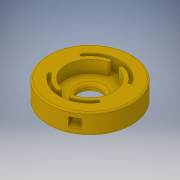
# Autodesk Inventor part: BasePaletas
Saved by Autodesk Inventor 2019 (Build 230136000, 136)
## iProperties
Created: 2019-12-12
Part Number: BasePaletas
Material: Generic
Document SubType Name: Modeling
Designer: Sergio
Density: 1 g/cm^3
Appearance: Gold
Author: Sergio
Autodesk Inventor part; units mm, degrees
ref_plane "XZ Plane" through (0, 0, 0) normal (0, 1, 0) x (-1, 0, 0)
sketch "Sketch3" plane through (0, 0, 0) normal (1, 0, 0) x (0, 1, 0)
  line L0 (63.5252, 0) -> (0, 0) construction
  line L1 (0, -7) -> (0, -27)
  line L2 (0, -27) -> (13, -27)
  line L3 (13, -27) -> (13, -15.23)
  line L4 (0, -7) -> (5, -7)
  line L5 (5, -7) -> (5, -15.23)
  line L6 (5, -15.23) -> (13, -15.23)
  dimension "d15" = 13
  dimension "d18" = 5
  dimension "d28" = 7
  dimension "d32" = 27
  dimension "d33" = 15.23
  constraints: 14 end point, 3 perpendicular, 2 horizontal, 1 coincident, 1 parallel, 1 vertical
  measures "d15" distance between parallel lines of L3 L1
  measures "d18" distance of L1.start L4.end
  measures "d28" distance between parallel lines of L4 L0
  measures "d32" distance between parallel lines of L0 L2
  measures "d33" distance between parallel lines of L0 L6
revolve "Revolution1" add sketch "Sketch3" angle 360 about axis through (0, 63.5252, 0) along (0, -1, 0)
fillet "Fillet2" radius 1 2 edges at (0, 13, 27) (0, 0, 27)
ref_plane "Work Plane2" through (-27, 6.5, 0) normal (1, 0, 0) x (0, 1, 0)
sketch "Sketch4" plane through (-27, 6.5, 0) normal (1, 0, 0) x (0, 1, 0)
  line L0 (-6.5, 0) -> (13.3256, 0) construction
  line L1 (-3.0202, 3.035) -> (3.0498, 3.035)
  line L2 (3.0498, 3.035) -> (3.0498, -3.035)
  line L3 (3.0498, -3.035) -> (-3.0202, -3.035)
  line L4 (-3.0202, -3.035) -> (-3.0202, 3.035)
  line L5 (-3.0202, 3.035) -> (3.0498, -3.035) construction
  line L6 (3.0498, 3.035) -> (-3.0202, -3.035) construction
  point P0 (0.0148, 0)
  dimension "d21" = 6.07
  dimension "d22" = 6.07
  constraints: 14 end point, 2 horizontal, 2 midpoint, 2 parallel, 1 perpendicular, 1 point on line
  measures "d21" distance of L2.end L3.end
  measures "d22" distance of L1.end L2.end
extrude "Extrusion3" cut sketch "Sketch4" along normal blind 10
pattern_circular "Circular Pattern2" count 3 over 360 about axis through (0, 9, 0) along (0, -1, 0) of "Extrusion3"
fillet "Fillet4" radius 2 1 edges at (0, 0, 7)
fillet "Fillet5" radius 2 1 edges at (0, 5, 7)
ref_plane "Work Plane3" through (0, 6.5, -27) normal (0, 0, 1) x (1, 0, 0)
sketch "Sketch5" plane through (0, 6.5, -27) normal (0, 0, 1) x (1, 0, 0)
  line L0 (27, 5.5) -> (-27, 5.5) projected
  line L1 (-3.7766, 5.5) -> (3.7234, 5.5)
  line L2 (3.7234, 5.5) -> (3.7234, 3.9)
  line L3 (3.7234, 3.9) -> (-3.7766, 3.9)
  line L4 (-3.7766, 3.9) -> (-3.7766, 5.5)
  line L5 (-0.0266, 2.2373) -> (-0.0266, 10.6054) construction
  point P0 (0, -6.5)
  dimension "d34" = 3.75
  dimension "d35" = 3.75
  dimension "d36" = 1.6
  constraints: 10 end point, 2 parallel, 1 horizontal, 1 perpendicular, 1 point on line, 1 vertical
  measures "d34" distance between parallel lines of L2 L5
  measures "d35" distance between parallel lines of L4 L5
  measures "d36" distance of L3.end L1.start
extrude "Extrusion4" cut sketch "Sketch5" along normal blind 7
sketch "Sketch7" plane through (0, 13, 0) normal (0, 1, 0) x (1, 0, 0)
  arc A0 (-13.8497, -9.3315) -> (13.8497, -9.3315) centre (0, 0) ccw
  arc A1 (-3.0841, -11.7521) -> (3.0841, -11.7521) centre (0, 0) ccw
  line L0 (0, 33.2339) -> (0, -33.2339) construction
  circle A2 centre (0, 0) radius 13.45 construction
  circle A3 centre (0, 0) radius 15.7 construction
  arc A4 (-3.3691, -14.3087) -> (-3.0841, -11.7521) centre (-3.4141, -13.0095) ccw
  arc A5 (3.0841, -11.7521) -> (3.7441, -14.2669) centre (3.4141, -13.0095) ccw
  arc A6 (-12.191, -8.2139) -> (-13.8497, -9.3315) centre (-13.0204, -8.7727) ccw
  arc A7 (13.8497, -9.3315) -> (12.399, -7.9891) centre (13.0204, -8.7727) ccw
  arc A8 (-12.191, -8.2139) -> (-3.3691, -14.3087) centre (0, 0) ccw
  arc A9 (3.7441, -14.2669) -> (12.399, -7.9891) centre (0, 0) ccw
  point P0 (0, 0)
  dimension "d42" = 26.9
  dimension "d43" = 31.4
  dimension "d40" = 33.4
  dimension "d41" = 24.3
  constraints: 16 point on circle, 8 centre point, 5 coincident, 2 end point, 2 symmetric about line, 1 tangent, 1 vertical, 8 other
  measures "d40" diameter of A0
  measures "d41" diameter of A1
sketch "Sketch8" plane through (0, 13, 0) normal (0, 1, 0) x (1, 0, 0)
  line L0 (0, 33.2339) -> (0, -33.2339) construction
  circle A0 centre (0, 0) radius 16.45 construction
  circle A1 centre (0, 0) radius 18.7 construction
  circle A2 centre (-4.1756, -15.9112) radius 1.25
  circle A3 centre (4.1756, -15.9112) radius 1.25
  circle A4 centre (-15.5083, -10.449) radius 1
  circle A5 centre (15.5083, -10.449) radius 1
  line L1 (-35.9812, 0) -> (51.1812, 0) construction
  arc A6 (-16.3377, 11.0078) -> (-14.679, 9.8902) centre (-15.5083, 10.449) ccw
  arc A7 (-3.8583, 14.7022) -> (-4.4929, 17.1203) centre (-4.1756, 15.9112) ccw
  arc A8 (4.4929, 17.1203) -> (3.8583, 14.7022) centre (4.1756, 15.9112) ccw
  arc A9 (14.679, 9.8902) -> (16.3377, 11.0078) centre (15.5083, 10.449) ccw
  arc A10 (3.8583, 14.7022) -> (-3.8583, 14.7022) centre (0, 0) ccw
  arc A11 (-3.8583, -14.7022) -> (3.8583, -14.7022) centre (0, 0) ccw
  arc A12 (-4.4929, 17.1203) -> (-14.679, 9.8902) centre (0, 0) ccw
  arc A13 (-17.7, 0) -> (17.7, 0) centre (0, 0) ccw
  arc A14 (14.679, 9.8902) -> (4.4929, 17.1203) centre (0, 0) ccw
  arc A15 (-19.7, 0) -> (19.7, 0) centre (0, 0) ccw
  arc A16 (16.3377, 11.0078) -> (-16.3377, 11.0078) centre (0, 0) ccw
  point P0 (0, 0)
  dimension "d48" = 32.9
  dimension "d49" = 37.4
  constraints: 22 point on circle, 13 centre point, 6 symmetric about line, 5 coincident, 4 end point, 4 point on line, 2 vertical, 1 horizontal, 17 other
extrude "Extrusion6" cut sketch "Sketch8" against normal blind 8 contours A16 A9 A14 A8 A10 A7 A12 A6
mirror "Mirror2" about plane through (0, 0, 0) normal (0, 0, 1) of "Extrusion6"
body "Solid2"
